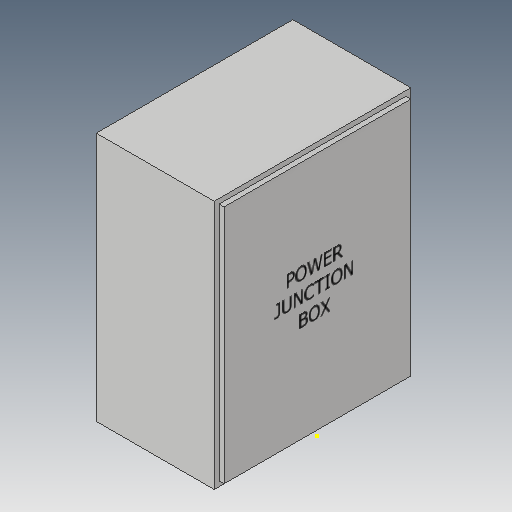
# Autodesk Inventor part: powerBox
Saved by Autodesk Inventor 2017 (Build 210142000, 142)
## iProperties
Created: 2016-08-11
Part Number: powerBox
Material: Generic
Document SubType Name: Modeling
Designer: Zara
Density: 1 g/cm^3
Appearance: Default
Author: Zara
Autodesk Inventor part; units mm, degrees
ref_plane "YZ Plane" through (0, 0, 0) normal (1, 0, 0) x (0, 1, 0)
ref_plane "XZ Plane" through (0, 0, 0) normal (0, 1, 0) x (-1, 0, 0)
ref_plane "XY Plane" through (0, 0, 0) normal (0, 0, 1) x (1, 0, 0)
sketch "Sketch1" plane through (0, 0, 0) normal (0, 1, 0) x (-1, 0, 0)
  line L0 (-120, 200) -> (120, 200)
  line L1 (120, 200) -> (120, -200)
  line L2 (120, -200) -> (-120, -200)
  line L3 (-120, -200) -> (-120, 200)
  line L4 (-120, 200) -> (120, -200) construction
  line L5 (120, 200) -> (-120, -200) construction
  point P0 (0, 0)
  dimension "d0" = 400
  dimension "d1" = 240
  constraints: 12 end point, 2 midpoint, 2 parallel, 1 horizontal, 1 perpendicular
  measures "d0" distance of L0.end L1.end
  measures "d1" distance of L1.end L2.end
extrude "Extrusion1" add sketch "Sketch1" along normal blind 508
sketch "Sketch2" plane through (0, 0, 0) normal (0, -1, 0) x (1, 0, 0)
  point P0 (0, 0)
sketch "Sketch3" plane through (0, 0, 0) normal (0, -1, 0) x (1, 0, 0)
  circle A0 centre (-40.68, 94.7135) radius 24.5
  circle A1 centre (-40.68, -105.2865) radius 24.5
  line L0 (-120, 200) -> (-120, -200) projected
  point P0 (0, 0)
  dimension "d4" = 49
  dimension "d5" = 49
  dimension "d6" = 200
  dimension "d17" = 79.32
  dimension "d18" = 79.32
  constraints: 2 centre point
  measures "d4" diameter of A0
  measures "d5" diameter of A1
  measures "d6" distance of A1.centre A0.centre
  measures "d17" distance from line of L0 A0.centre
  measures "d18" distance from line of L0 A1.centre
shell "Shell1" thickness 10 removed faces 0
extrude "Extrusion2" cut sketch "Sketch3" against normal blind 10
sketch "Sketch4" plane through (120, 0, 200) normal (1, 0, 0) x (0, 0, -1)
  line L0 (10, 498) -> (390, 498) projected
  line L1 (390, 10) -> (390, 498) projected
  line L2 (10, 498) -> (390, 498)
  line L3 (390, 498) -> (390, 10)
  line L4 (390, 10) -> (10, 10)
  line L5 (10, 10) -> (10, 498)
  point P0 (200, 0)
  constraints: 8 end point, 2 parallel, 1 horizontal, 1 perpendicular
extrude "Extrusion3" add sketch "Sketch4" along normal blind 10
sketch "Sketch5" plane through (130, 0, 200) normal (1, 0, 0) x (0, 0, -1)
  line L0 (112.0478, 315.562) -> (275.2746, 315.562) construction
  line L1 (275.2746, 315.562) -> (275.2746, 205.4508) construction
  line L2 (275.2746, 205.4508) -> (112.0478, 205.4508) construction
  line L3 (112.0478, 205.4508) -> (112.0478, 315.562) construction
  point P0 (200, 0)
  constraints: 2 other
body "Solid1"
